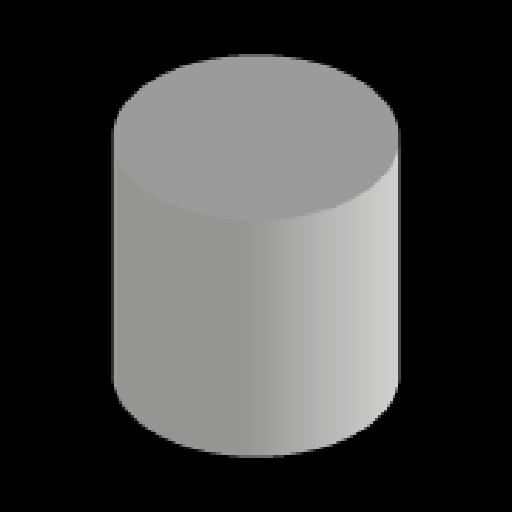
# Autodesk Inventor part: CartWheelCap
Saved by Autodesk Inventor 2025 (Build 290162000, 162)
## iProperties
Created: 2025-03-06
Part Number: CartWheelCap
Material: Generic
Document SubType Name: Modeling
Designer: Trevor
Density: 1 g/cm^3
Appearance: Default
Author: Trevor
Autodesk Inventor part; units mm, degrees
ref_plane "YZ Plane" through (0, 0, 0) normal (1, 0, 0) x (0, 1, 0)
ref_plane "XZ Plane" through (0, 0, 0) normal (0, 1, 0) x (-1, 0, 0)
ref_plane "XY Plane" through (0, 0, 0) normal (0, 0, 1) x (1, 0, 0)
sketch "Sketch1" plane through (0, 0, 0) normal (0, 0, 1) x (1, 0, 0)
  circle A0 centre (0, 0) radius 6.35 projected
  circle A1 centre (0, 0) radius 3.175 projected
  circle A2 centre (0, 0) radius 2.975
  point P0 (0, 0)
  dimension "d0" = 0.2
  constraints: 1 centre point
  measures "d0" radial gap between concentric circles of A1 A2
extrude "Extrusion1" add sketch "Sketch1" against normal blind 6 contours A2
sketch "Sketch2" plane through (0, 0, 0) normal (0, 0, 1) x (1, 0, 0)
  circle A0 centre (0, 0) radius 2.975 projected
  point P0 (0, 0)
extrude "Extrusion2" add sketch "Sketch2" along normal blind 0.2
sketch "Sketch3" plane through (0, 0, 0.2) normal (0, 0, 1) x (1, 0, 0)
  circle A0 centre (0, 0) radius 6.75 projected
  circle A1 centre (0, 0) radius 19.05 projected
  circle A2 centre (0, 0) radius 8.75
  point P0 (0, 0)
  dimension "d5" = 2
  constraints: 1 centre point
  measures "d5" radial gap between concentric circles of A0 A2
extrude "Extrusion3" add sketch "Sketch3" along normal blind 1 contours A0 | A2
body "Solid1"
